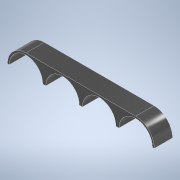
# Autodesk Inventor part: batteryspacer
Saved by Autodesk Inventor 2022 (Build 260153000, 153)
## iProperties
Created: 2021-10-06
Part Number: batteryspacer
Material: Generic
Document SubType Name: Modeling
Designer: Bowen O'Steen
Density: 1 g/cm^3
Appearance: Dark Gray
Author: Bowen O'Steen
Autodesk Inventor part; units mm, degrees
ref_plane "YZ Plane" through (0, 0, 0) normal (1, 0, 0) x (0, 1, 0)
ref_plane "XZ Plane" through (0, 0, 0) normal (0, 1, 0) x (-1, 0, 0)
ref_plane "XY Plane" through (0, 0, 0) normal (0, 0, 1) x (1, 0, 0)
sketch "Sketch1" plane through (0, 0, 0) normal (0, 0, 1) x (1, 0, 0)
  circle A0 centre (0, 0) radius 9.165
  line L0 (0, 0) -> (-2.3778, 0) construction
  circle A1 centre (-20, 0) radius 9.165
  circle A2 centre (-40, 0) radius 9.165
  circle A3 centre (-60, 0) radius 9.165
  arc A4 (10.165, 0) -> (0, 10.165) centre (0, 0) ccw
  arc A5 (-60, 10.165) -> (-70.165, 0) centre (-60, 0) ccw
  line L1 (-60, 10.165) -> (0, 10.165)
  line L2 (-50.835, 0) -> (-49.165, 0)
  line L3 (-30.835, 0) -> (-29.165, 0)
  line L4 (-10.835, 0) -> (-9.165, 0)
  line L5 (-70.165, 0) -> (-69.165, 0)
  line L6 (9.165, 0) -> (10.165, 0)
  dimension "d0" = 18.33
  dimension "d3" = 20
  dimension "d8" = 1
  dimension "d9" = 1
  constraints: 14 end point, 12 point on circle, 6 centre point, 6 point on line, 4 horizontal, 1 coincident, 1 tangent, 6 other
  measures "d0" diameter of A0
  measures "d3" distance of L0.start A1.centre
  measures "d8" radial gap between concentric circles of A0 A4
  measures "d9" radial gap between concentric circles of A3 A5
extrude "Extrusion1" add sketch "Sketch1" along normal mid plane 10 contours A0 L4 A1 L3 A2 L2 A3 L5 A5 L1 A4 L6
body "Solid1"
